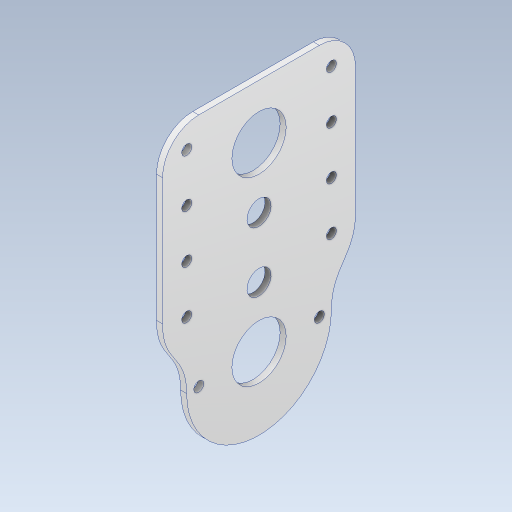
# Autodesk Inventor part: L1Plate
Saved by Autodesk Inventor 2023 (Build 270158000, 158)
## iProperties
Created: 2023-02-05
Part Number: L1Plate
Material: Aluminum 6061
Document SubType Name: Modeling
Designer: Dave
Density: 2.7 g/cm^3
Appearance: Aluminum - Flat
Mass: 543.403 g
Surface Area: 1367.92 cm^2
Volume: 201.26 cm^3
Author: Dave
Autodesk Inventor part; units mm, degrees
ref_plane "YZ Plane" through (0, 0, 0) normal (1, 0, 0) x (0, 1, 0)
ref_plane "XZ Plane" through (0, 0, 0) normal (0, 1, 0) x (-1, 0, 0)
ref_plane "XY Plane" through (0, 0, 0) normal (0, 0, 1) x (1, 0, 0)
sketch "Sketch1" plane through (0, 0, 0) normal (1, 0, 0) x (0, 1, 0)
  line L0 (0, 0) -> (101.6, 0)
  line L1 (101.6, 0) -> (101.6, -152.4)
  line L2 (101.6, -152.4) -> (0, -152.4)
  line L3 (0, -152.4) -> (0, 0)
  circle A0 centre (50.8, -28.575) radius 14.2875
  circle A1 centre (50.8, -60.325) radius 6.35
  circle A2 centre (50.8, -92.075) radius 6.35
  circle A3 centre (50.8, -123.825) radius 14.2875
  line L4 (50.8, -28.575) -> (50.8, -123.825) construction
  circle A4 centre (88.9, -12.7) radius 2.65
  circle A5 centre (88.9, -38.1) radius 2.65
  circle A6 centre (88.9, -63.5) radius 2.65
  circle A7 centre (88.9, -88.9) radius 2.65
  circle A8 centre (88.9, -114.3) radius 2.65
  circle A9 centre (88.9, -139.7) radius 2.65
  circle A10 centre (12.7, -12.7) radius 2.65
  circle A11 centre (12.7, -38.1) radius 2.65
  circle A12 centre (12.7, -63.5) radius 2.65
  circle A13 centre (12.7, -88.9) radius 2.65
  circle A14 centre (12.7, -114.3) radius 2.65
  circle A15 centre (12.7, -139.7) radius 2.65
  line L5 (76.2, -152.4) -> (76.2, -508.635)
  line L6 (25.4, -187.175) -> (25.4, -152.4)
  circle A16 centre (50.8, -212.575) radius 6.35
  line L7 (50.8, -212.575) -> (-444.4159, 282.6409) construction
  line L8 (50.8, -212.575) -> (751.141, -212.575) construction
  line L9 (-161.775, -263.375) -> (-9.375, -263.375)
  line L10 (-9.375, -263.375) -> (-9.375, -161.775)
  line L11 (-9.375, -161.775) -> (-161.775, -161.775)
  circle A17 centre (-133.2, -212.575) radius 14.2875
  circle A18 centre (-101.45, -212.575) radius 6.35
  circle A19 centre (-69.7, -212.575) radius 6.35
  circle A20 centre (-37.95, -212.575) radius 14.2875
  line L12 (-133.2, -212.575) -> (-37.95, -212.575) construction
  circle A21 centre (-149.075, -250.675) radius 2.65
  circle A22 centre (-123.675, -250.675) radius 2.65
  circle A23 centre (-98.275, -250.675) radius 2.65
  circle A24 centre (-72.875, -250.675) radius 2.65
  circle A25 centre (-47.475, -250.675) radius 2.65
  circle A26 centre (-22.075, -250.675) radius 2.65
  circle A27 centre (-149.075, -174.475) radius 2.65
  circle A28 centre (-123.675, -174.475) radius 2.65
  circle A29 centre (-98.275, -174.475) radius 2.65
  circle A30 centre (-72.875, -174.475) radius 2.65
  circle A31 centre (-47.475, -174.475) radius 2.65
  circle A32 centre (-22.075, -174.475) radius 2.65
  line L13 (-9.375, -237.975) -> (346.86, -237.975)
  line L14 (25.4, -187.175) -> (-9.375, -187.175)
  circle A33 centre (50.8, -212.575) radius 6.35
  line L15 (50.8, -212.575) -> (50.8, -912.916) construction
  line L16 (76.2, -237.975) -> (346.86, -237.975)
  line L17 (76.2, -508.635) -> (76.2, -237.975)
  line L18 (-161.775, -161.775) -> (-161.775, -263.375)
  circle A34 centre (50.8, -28.575) radius 25.4 construction
  circle A35 centre (50.8, -28.575) radius 38.1
  circle A36 centre (82.55, -28.575) radius 2.65
  circle A37 centre (19.05, -28.575) radius 2.65
  line L19 (88.9, -28.575) -> (88.9, -47.625) construction
  line L20 (88.9, -47.625) -> (101.6, -47.625) construction
  line L21 (101.6, -47.625) -> (101.6, -66.675) construction
  spline S0 degree 3 poles (88.9, -28.575) (88.9, -47.625) (101.6, -47.625) (101.6, -66.675) knots 1 1 1 1 2 2 2 2
  line L22 (12.7, -28.575) -> (12.7, -47.625) construction
  line L23 (12.7, -47.625) -> (0, -47.625) construction
  line L24 (0, -47.625) -> (0, -66.675) construction
  spline S1 degree 3 poles (12.7, -28.575) (12.7, -47.625) (0, -47.625) (0, -66.675) knots 1 1 1 1 2 2 2 2
  spline S2 degree 3 poles (-133.2, -174.475) (-114.15, -174.475) (-114.15, -161.775) (-95.1, -161.775) knots 1 1 1 1 2 2 2 2
  line L25 (-133.2, -174.475) -> (-114.15, -174.475) construction
  line L26 (-114.15, -174.475) -> (-114.15, -161.775) construction
  line L27 (-114.15, -161.775) -> (-95.1, -161.775) construction
  circle A38 centre (-133.2, -212.575) radius 38.1
  circle A39 centre (-133.2, -180.825) radius 2.65
  spline S3 degree 3 poles (-133.2, -250.675) (-114.15, -250.675) (-114.15, -263.375) (-95.1, -263.375) knots 1 1 1 1 2 2 2 2
  line L28 (-133.2, -250.675) -> (-114.15, -250.675) construction
  line L29 (-114.15, -250.675) -> (-114.15, -263.375) construction
  line L30 (-114.15, -263.375) -> (-95.1, -263.375) construction
  circle A40 centre (-133.2, -244.325) radius 2.65
  point P0 (101.6, -76.2)
  point P1 (50.8, -76.2)
  point P2 (50.8, -152.4)
  point P3 (-85.575, -263.375)
  point P4 (-85.575, -212.575)
  point P5 (-9.375, -212.575)
  point P6 (63.5, -470.535)
  point P7 (0, -66.675)
  point P8 (-126.2384, -251.347)
  point P9 (-121.9095, -252.6512)
  dimension "d32" = 76.2
  dimension "d0" = 101.6
  dimension "d1" = 152.4
  dimension "d2" = 28.575
  dimension "d3" = 12.7
  dimension "d4" = 12.7
  dimension "d5" = 28.575
  dimension "d6" = 31.75
  dimension "d7" = 31.75
  dimension "d8" = 31.75
  dimension "d9" = 5.3
  dimension "d10" = 12.7
  dimension "d11" = 12.7
  dimension "d14" = 25.4
  dimension "d17" = 76.2
  dimension "d22" = 12.7
  dimension "d24" = 184
  dimension "d25" = 25.4
  dimension "d26" = 50.8
  dimension "d27" = 135
  dimension "d31" = 50.8
  dimension "d33" = 31.75
  dimension "d34" = 31.75
  dimension "d35" = 19.05
  dimension "d36" = 19.05
  dimension "d39" = 90
  dimension "d41" = 31.75
  constraints: 39 centre point, 38 end point, 31 symmetric about line, 9 point on line, 5 horizontal, 5 vertical, 5 vertical alignment, 3 equal radius, 3 horizontal alignment, 3 midpoint, 3 perpendicular, 2 coincident, 2 parallel, 1 equal length, 78 other
  measures "d0" distance of L1.end L2.end
  measures "d1" distance of L0.end L1.end
  measures "d2" diameter of A0
  measures "d3" diameter of A1
  measures "d4" diameter of A2
  measures "d5" diameter of A3
  measures "d6" distance of A1.centre L4.start
  measures "d7" distance of A2.centre A1.centre
  measures "d8" distance of A2.centre L4.end
  measures "d9" diameter of A4
  measures "d10" distance from line of L1 A4.centre
  measures "d11" distance from line of L0 A4.centre
  measures "d14" distance of A4.centre A5.centre
  measures "d17" distance of A4.centre A10.centre
  measures "d22" diameter of A16
  measures "d24" distance of L7.start L4.start
  measures "d25" distance between parallel lines of L4 L5
  measures "d26" distance between parallel lines of L5 L6
  measures "d27" angle of L8 L7
  measures "d31" diameter of A34
  measures "d33" distance of A36.centre A34.centre
  measures "d34" distance of L4.start A37.centre
  measures "d35" distance of L19.start L19.end
  measures "d36" distance of L21.end L20.end
  measures "d41" distance of A40.centre L12.start
extrude "Extrusion1" add sketch "Sketch1" along normal blind 3.175 contours L10 L9 S3 A22 A38 A28 S2 L11 | A28 A38 S2 | S3 A22 A38 | A38 A28 A22 L18 | L18 A38 | A28 A38 S2 | S3 A38 A22 | A28 A38 | A22 A38
fillet "Fillet1" [suppressed]
fillet "Fillet2" [suppressed]
fillet "Fillet3" radius 19.05 2 edges at (1.5875, -9.375, -161.775) (1.5875, -9.375, -263.375)
equation "\"d7\" = d6"
equation "\"d8\" = d7"
body "Solid1"
